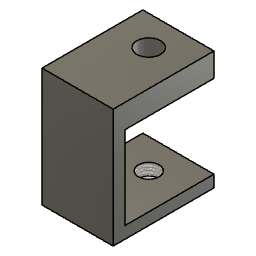
Replace base v4 (Autodesk Fusion 360 design; units mm, degrees)
Autodesk Fusion 360 part; units mm, degrees
sketch "草图1" plane through (0, 0, 0) normal (0, 1, 0) x (1, 0, 0) in component "Component"
  line L0 (-30, 25) -> (30, 25)
  line L1 (30, 25) -> (30, -60)
  line L2 (30, -60) -> (-30, -60)
  line L3 (-30, -60) -> (-30, 25)
  dimension "d1" = 60
  dimension "d2" = 85
  dimension "d3" = 25
  dimension "d4" = 30
  constraint horizontal L0
  constraint vertical L1
  constraint horizontal L2
  constraint vertical L3
  measures "d1" distance of L0.start L0.end
  measures "d2" distance of L0.start L2.end
  measures "d3" distance of origin L0
  measures "d4" distance of origin L3
extrude "拉伸1" add sketch "草图1" along normal blind 10 in component "Component"
sketch "草图2" plane through (0, 0, 0) normal (0, -1, 0) x (1, 0, 0) in component "Component"
  line L0 (30, 60) -> (-30, 60)
  line L1 (-30, 60) -> (-30, -25)
  line L2 (-30, -25) -> (30, -25)
  line L3 (30, -25) -> (30, 60)
  line L4 (-30, 60) -> (30, 60)
  line L5 (30, 60) -> (30, 50)
  line L6 (30, 50) -> (-30, 50)
  line L7 (-30, 50) -> (-30, 60)
  dimension "d8" = 10
  constraint horizontal L4
  constraint vertical L5
  constraint horizontal L6
  constraint vertical L7
  constraint coincident L3 L5.end
  constraint coincident L0.end L1.start
  measures "d8" distance of L0.end L6.end
extrude "拉伸2" add sketch "草图2" along normal blind 80 contours L0 L1 L3 L4 L5 L6 L7 in component "Component"
sketch "草图3" plane through (0, 0, 50) normal (0, 0, -1) x (-1, 0, 0) in component "Component"
  line L0 (30, 0) -> (-30, 0)
  line L1 (-30, 0) -> (-30, -80)
  line L2 (-30, -80) -> (30, -80)
  line L3 (30, -80) -> (30, 0)
  line L4 (-30, -70) -> (30, -70)
  line L5 (30, -70) -> (30, -80)
  line L6 (30, -80) -> (-30, -80)
  line L7 (-30, -80) -> (-30, -70)
  dimension "d11" = 10
  constraint horizontal L4
  constraint vertical L5
  constraint horizontal L6
  constraint vertical L7
  constraint coincident L2.end L3.start
  constraint coincident L1 L4.start
  measures "d11" distance of L4.start L1.end
extrude "拉伸3" add sketch "草图3" along normal blind 75 contours L1 L2 L3 L4 L5 L6 L7 in component "Component"
sketch "草图4" plane through (0, -80, 0) normal (0, -1, 0) x (1, 0, 0) in component "Component"
  line L0 (30, -25) -> (30, 60)
  line L1 (30, 60) -> (-30, 60)
  line L2 (-30, 60) -> (-30, -25)
  line L3 (-30, -25) -> (30, -25)
  circle A0 centre (0, 0) radius 10
  dimension "d14" = 20
  constraint coincident A0.centre origin
  measures "d14" diameter of A0
extrude "拉伸4" cut sketch "草图4" against normal blind 10 contours A0 in component "Component"
thread "螺纹1" "ISO Metric profile 20.0 M20x2.5 6H" major diameter 20.2925 minor diameter 17.519 pitch 2.5 angle 60 resizes the face on face at (9.9876, -73.3333, -0.4985) in component "Component"
extrude "拉伸5" add 1 faces at (-10, 10, 3.3333) along direction (0, 1, 0) blind 10 in component "Component"
sketch "草图5" plane through (0, 20, 0) normal (0, 1, 0) x (-1, 0, 0) in component "Component"
  line L0 (30, 60) -> (-30, 60)
  line L1 (-30, 60) -> (-30, -25)
  line L2 (-30, -25) -> (30, -25)
  line L3 (30, -25) -> (30, 60)
  circle A0 centre (0, 0) radius 10
  constraint coincident A0.centre origin
extrude "拉伸6" cut sketch "草图5" against normal blind 15 contours A0 in component "Component"
component "Component" placed x (1, 0, 0) y (0, 1, 0) z (0, 0, 1) at (0, 0, 0)
